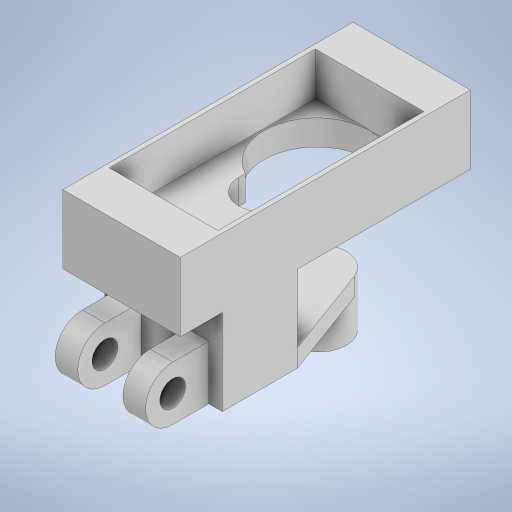
# Autodesk Inventor part: ServoMount
Saved by Autodesk Inventor 2023 (Build 270158000, 158)
## iProperties
Created: 2022-10-13
Part Number: ServoMount
Material: Generic
Document SubType Name: Modeling
Designer: GROS
Density: 1 g/cm^3
Appearance: Default
Author: GROS
Autodesk Inventor part; units mm, degrees
ref_plane "YZ Plane" through (0, 0, 0) normal (1, 0, 0) x (0, 1, 0)
ref_plane "XZ Plane" through (0, 0, 0) normal (0, 1, 0) x (-1, 0, 0)
ref_plane "XY Plane" through (0, 0, 0) normal (0, 0, 1) x (1, 0, 0)
sketch "Sketch1" plane through (0, 0, 0) normal (0, 1, 0) x (-1, 0, 0)
  line L0 (0, 0) -> (12, 0)
  line L1 (12, 0) -> (12, -22.8)
  line L2 (12, -22.8) -> (0, -22.8)
  line L3 (0, -22.8) -> (0, 0)
  line L4 (6, -22.8) -> (6, -11.1)
  line L5 (12, 0) -> (12, 4.65)
  line L6 (12, 4.65) -> (12.5, 4.65)
  line L7 (0, -22.8) -> (-0.5, -22.8)
  line L8 (-0.5, -22.8) -> (-0.5, -27.45)
  line L9 (12.5, 4.65) -> (-0.5, 4.65)
  line L10 (-0.5, 4.65) -> (-0.5, -27.45)
  line L11 (-0.5, -27.45) -> (12.5, -27.45)
  line L12 (12.5, -27.45) -> (12.5, 4.65)
  circle A0 centre (6, -16.95) radius 5.85
  line L13 (6, -11.1) -> (6, -8.3)
  line L14 (6, -8.3) -> (6, -11.05)
  circle A1 centre (6, -11.05) radius 2.75
  line L15 (3.25, -11.05) -> (3.25, -11.7867)
  line L16 (8.75, -11.05) -> (8.75, -11.7867)
  dimension "d0" = 22.8
  dimension "d1" = 12
  dimension "d5" = 4.65
  dimension "d6" = 0.5
  dimension "d7" = 0.5
  dimension "d8" = 4.65
  dimension "d42" = 11.7
  dimension "d43" = 2.8
  dimension "d44" = 2.75
  constraints: 34 end point, 6 point on circle, 5 parallel, 5 vertical, 4 horizontal, 2 centre point, 2 midpoint, 2 perpendicular, 2 tangent, 1 coincident, 1 point on line
  measures "d0" distance of L0.end L1.end
  measures "d1" distance of L0.start L0.end
  measures "d5" distance of L0.end L5.end
  measures "d6" distance of L5.end L6.end
  measures "d7" distance of L2.end L7.end
  measures "d8" distance of L7.end L8.end
  measures "d42" distance of L4.start L4.end
  measures "d43" distance of L4.end L13.end
  measures "d44" distance of L13.end L14.end
extrude "Extrusion1" add sketch "Sketch1" along normal blind 2.8 contours L0 L1 L2 L3
extrude "Extrusion3" add sketch "Sketch1" along normal blind 7.6 contours L3 L7 L10 L9 L5 L0 | L5 L6 L12 L11 L8 L7 L2 L1
sketch "Sketch5" plane through (0, 0, 0) normal (0, -1, 0) x (1, 0, 0)
  line L0 (0.5, 4.65) -> (0.5, -27.45) projected
  line L1 (0.5, 4.65) -> (0.5, 0)
  line L2 (-12.5, -27.45) -> (-12.5, 4.65) projected
  line L3 (0.5, 0) -> (-12.5, 0)
  line L4 (-12.5, 0) -> (-12.5, -8.3)
  line L5 (-12.5, -8.3) -> (0.5, -8.3)
  line L6 (0.5, -8.3) -> (0.5, 0)
  point P0 (0, 0)
  dimension "d45" = 4.65
  dimension "d46" = 8.3
  constraints: 10 end point, 2 parallel, 2 point on line, 1 horizontal, 1 perpendicular
  measures "d45" distance of L0.start L1.end
  measures "d46" distance of L3.end L4.end
extrude "Extrusion8" add sketch "Sketch5" along normal blind 7.5
sketch "Sketch6" plane through (0, -7.5, 0) normal (0, -1, 0) x (1, 0, 0)
  line L0 (-6, -22.8) -> (-12, -22.8) projected
  line L1 (-6, -22.8) -> (-6, -17.2)
  circle A0 centre (-6, -17.2) radius 3.025
  line L2 (0.5, 0) -> (-12.5, 0) projected
  line L3 (-6, -8.3) -> (-12.5, -8.3) projected
  line L4 (0.5, 0) -> (-12.5, 0)
  line L5 (-12.5, 0) -> (-12.5, -8.3)
  line L6 (-12.5, -8.3) -> (0.5, -8.3)
  line L7 (0.5, -8.3) -> (0.5, 0)
  line L8 (-12.5, -8.3) -> (-7.8416, -20.9536)
  line L9 (0.5, -8.3) -> (-6, -8.3) projected
  line L10 (0.5, -8.3) -> (-4.2111, -21.0966)
  point P0 (0, 0)
  point P1 (-12.5, 0)
  point P2 (-8.8387, -18.2451)
  point P3 (-3.1613, -18.2451)
  dimension "d49" = 5.6
  dimension "d50" = 6.05
  constraints: 14 end point, 2 parallel, 2 tangent, 1 centre point, 1 coincident, 1 horizontal, 1 perpendicular, 1 vertical
  measures "d49" distance of L0.start L1.end
  measures "d50" diameter of A0
extrude "Extrusion9" add sketch "Sketch6" along normal blind 2
sketch "Sketch7" plane through (0, -9.5, 0) normal (0, -1, 0) x (1, 0, 0)
  arc A0 (-8.75, -11.7867) -> (-3.25, -11.7867) centre (-6, -16.95) ccw projected
  line L0 (-6, -22.8) -> (-6, -17.2)
  circle A1 centre (-6, -17.2) radius 3.025
  point P0 (0, 0)
  dimension "d53" = 5.6
  dimension "d54" = 6.05
  constraints: 2 end point, 1 centre point, 1 coincident, 1 point on circle, 1 vertical
  measures "d53" distance of L0.start L0.end
  measures "d54" diameter of A1
extrude "Extrusion10" add sketch "Sketch7" along normal blind 4
sketch "Sketch8" plane through (-12.5, 0, 0) normal (0, 0, 1) x (1, 0, 0)
  line L0 (13, -9.5) -> (0, -9.5) projected
  line L1 (6.5, -9.5) -> (9, -9.5)
  line L2 (6.5, -9.5) -> (4, -9.5)
  line L3 (9, -9.5) -> (11.5, -9.5)
  line L4 (11.5, -9.5) -> (11.5, -3.5)
  line L5 (11.5, -3.5) -> (9, -3.5)
  line L6 (9, -3.5) -> (9, -9.5)
  line L7 (4, -9.5) -> (1.5, -9.5)
  line L8 (1.5, -9.5) -> (1.5, -3.5)
  line L9 (1.5, -3.5) -> (4, -3.5)
  line L10 (4, -3.5) -> (4, -9.5)
  point P0 (12.5, 0)
  point P1 (1.5, -9.5)
  dimension "d58" = 2.5
  dimension "d59" = 2.5
  dimension "d60" = 6
  dimension "d61" = 6
  dimension "d62" = 2.5
  dimension "d63" = 2.5
  constraints: 20 end point, 4 parallel, 3 midpoint, 2 horizontal, 2 perpendicular, 2 point on line
  measures "d58" distance of point (6.5, -9.5) L1.end
  measures "d59" distance of point (6.5, -9.5) L2.end
  measures "d60" distance of L9.end L2.end
  measures "d61" distance of L5.end L1.end
  measures "d62" distance of L4.end L5.end
  measures "d63" distance of L8.end L9.end
extrude "Extrusion11" add sketch "Sketch8" along normal blind 7
sketch "Sketch9" plane through (-11, -9.5, 0) normal (-1, 0, 0) x (0, 0, 1)
  line L0 (7, 6) -> (7, 0) projected
  line L1 (7, 3) -> (4, 3)
  circle A0 centre (4, 3) radius 3
  circle A1 centre (4, 3) radius 1.425
  line L2 (0, 6) -> (7, 6) projected
  line L3 (0, 0) -> (7, 0) projected
  line L4 (7, 6) -> (1.6009, 6)
  line L5 (1.6009, 6) -> (1.6009, 0)
  line L6 (1.6009, 0) -> (7, 0)
  line L7 (7, 0) -> (7, 6)
  point P0 (0, 9.5)
  point P1 (4, 6)
  point P2 (4, 0)
  dimension "d66" = 2.85
  dimension "d67" = 3
  constraints: 10 end point, 2 coincident, 2 horizontal, 2 parallel, 1 centre point, 1 midpoint, 1 perpendicular, 1 point on line, 3 other
  measures "d66" diameter of A1
  measures "d67" distance of L1.start L1.end
extrude "Extrusion12" cut sketch "Sketch9" against normal through all contours L0 A0 L2 | A1 | L0 L3 A0
body "Solid1"
